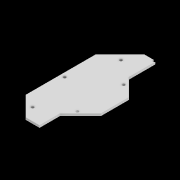
# Autodesk Inventor part: Placa Volante
Saved by Autodesk Inventor 2020 (Build 240168000, 168)
## iProperties
Created: 2022-11-26
Part Number: Placa Volante
Material: Genérico
Document SubType Name: Modeling
Designer: Alférez
Density: 1 g/cm^3
Appearance: Valor por defecto
Author: Alférez
Autodesk Inventor part; units mm, degrees
ref_plane "YZ Plane" through (0, 0, 0) normal (1, 0, 0) x (0, 1, 0)
ref_plane "XZ Plane" through (0, 0, 0) normal (0, 1, 0) x (-1, 0, 0)
ref_plane "XY Plane" through (0, 0, 0) normal (0, 0, 1) x (1, 0, 0)
sketch "Boceto1" plane through (0, 0, 0) normal (0, 1, 0) x (-1, 0, 0)
  line L0 (78, -28.2843) -> (49.7157, 0)
  line L1 (78, -129.6447) -> (42.6447, -165)
  line L2 (49.7157, 0) -> (29.7157, 0)
  line L3 (29.7157, 0) -> (29.7157, -30)
  line L4 (29.7157, -30) -> (0, -59.7157)
  line L5 (0, -59.7157) -> (0, -99.7157)
  line L6 (0, -99.7157) -> (25.4558, -125.1716)
  line L7 (0, -99.7157) -> (36, -99.7157) construction
  line L8 (78, -28.2843) -> (78, -129.6447)
  circle A0 centre (72, -78.6447) radius 2
  circle A1 centre (19.7157, -45) radius 2
  circle A2 centre (19.7157, -112) radius 2
  circle A3 centre (57.4939, -17.6777) radius 2
  circle A4 centre (52.5442, -140.9584) radius 2
  arc A5 (29.1447, -165) -> (25.4558, -163.5) centre (27.3714, -164.0751) ccw
  line L9 (29.1447, -165) -> (42.6447, -165)
  line L10 (25.4558, -125.1716) -> (25.4558, -163.5)
  point P0 (0, 0)
  dimension "d7" = 20
  dimension "d8" = 30
  dimension "d9" = 135
  dimension "d10" = 40
  dimension "d16" = 36
  dimension "d17" = 45
  dimension "d20" = 4
  dimension "d23" = 4
  dimension "d27" = 4
  dimension "d30" = 4
  dimension "d33" = 4
  dimension "d34" = 13.5
  constraints: 22 end point, 6 centre point, 2 horizontal, 2 point on circle, 1 equal length, 1 perpendicular, 1 vertical
  measures "d7" distance of L0.end L2.end
  measures "d8" distance of L2.end L3.end
  measures "d9" angle of L3 L4
  measures "d10" distance of L4.end L5.end
  measures "d16" distance of L5.end L6.end
  measures "d17" angle of L6 L7
  measures "d20" diameter of A0
  measures "d23" diameter of A1
  measures "d27" diameter of A2
  measures "d30" diameter of A3
  measures "d33" diameter of A4
  measures "d34" distance of L9.start L1.end
extrude "Extrusión1" add sketch "Boceto1" along normal blind 3
